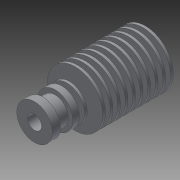
# Autodesk Inventor part: E3D_Chamber
Saved by Autodesk Inventor 2014 (Build 180170000, 170)
## iProperties
Created: 2014-09-30
Part Number: E3D_Chamber
Material: Generic
Document SubType Name: Modeling
Designer: ThatOtherGuy
Density: 1 g/cm^3
Appearance: Default
Author: ThatOtherGuy
Autodesk Inventor part; units mm, degrees
ref_plane "YZ Plane" through (0, 0, 0) normal (1, 0, 0) x (0, 1, 0)
ref_plane "XZ Plane" through (0, 0, 0) normal (0, 1, 0) x (-1, 0, 0)
ref_plane "XY Plane" through (0, 0, 0) normal (0, 0, 1) x (1, 0, 0)
sketch "Sketch1" plane through (0, 0, 0) normal (0, 0, 1) x (1, 0, 0)
  line L0 (0, 0) -> (0, 50.1)
  line L1 (8, 0) -> (8, 3.7)
  line L2 (8, 3.7) -> (6, 3.7)
  line L3 (6, 3.7) -> (6, 9.3)
  line L4 (6, 9.3) -> (8, 9.3)
  line L5 (8, 9.3) -> (8, 12.3)
  line L6 (8, 12.3) -> (4.5, 12.3)
  line L7 (4.5, 12.3) -> (4.5, 14.6)
  line L8 (4.5, 14.6) -> (8, 14.6)
  line L9 (8, 14.6) -> (8, 15.8)
  line L10 (8, 15.8) -> (4.5, 15.8)
  line L11 (4.5, 15.8) -> (4.5, 18.3)
  line L12 (4.5, 18.3) -> (12.5, 18.3)
  line L13 (12.5, 18.3) -> (12.5, 19.5)
  line L14 (12.5, 19.5) -> (4.5, 19.5)
  line L15 (4.5, 19.5) -> (4.5, 21.7)
  line L16 (4.5, 21.7) -> (12.5, 21.7)
  line L17 (12.5, 21.7) -> (12.5, 22.9)
  line L18 (12.5, 22.9) -> (4.5, 22.9)
  line L19 (4.5, 22.9) -> (4.5, 25.1)
  line L20 (4.5, 25.1) -> (12.5, 25.1)
  line L21 (12.5, 25.1) -> (12.5, 26.3)
  line L22 (12.5, 26.3) -> (4.5, 26.3)
  line L23 (4.5, 26.3) -> (4.5, 28.5)
  line L24 (4.5, 28.5) -> (12.5, 28.5)
  line L25 (12.5, 28.5) -> (12.5, 29.7)
  line L26 (12.5, 29.7) -> (6.5, 29.7)
  line L27 (6.5, 29.7) -> (6.5, 31.9)
  line L28 (6.5, 31.9) -> (12.5, 31.9)
  line L29 (12.5, 31.9) -> (12.5, 33.1)
  line L30 (12.5, 33.1) -> (7.5, 33.1)
  line L31 (7.5, 33.1) -> (7.5, 35.3)
  line L32 (7.5, 35.3) -> (12.5, 35.3)
  line L33 (12.5, 35.3) -> (12.5, 36.5)
  line L34 (12.5, 36.5) -> (7.5, 36.5)
  line L35 (7.5, 36.5) -> (7.5, 38.7)
  line L36 (7.5, 38.7) -> (12.5, 38.7)
  line L37 (12.5, 38.7) -> (12.5, 39.9)
  line L38 (12.5, 39.9) -> (7.5, 39.9)
  line L39 (7.5, 39.9) -> (7.5, 42.1)
  line L40 (7.5, 42.1) -> (12.5, 42.1)
  line L41 (12.5, 42.1) -> (12.5, 43.3)
  line L42 (12.5, 43.3) -> (7.5, 43.3)
  line L43 (7.5, 43.3) -> (7.5, 45.5)
  line L44 (7.5, 45.5) -> (12.5, 45.5)
  line L45 (12.5, 45.5) -> (12.5, 46.7)
  line L46 (12.5, 46.7) -> (7.5, 46.7)
  line L47 (7.5, 46.7) -> (7.5, 48.9)
  line L48 (7.5, 48.9) -> (12.5, 48.9)
  line L49 (12.5, 48.9) -> (12.5, 50.1)
  line L50 (12.5, 50.1) -> (3, 50.1)
  line L51 (3, 50.1) -> (3, 32.1)
  line L52 (3, 32.1) -> (1, 31.1)
  line L53 (1, 31.1) -> (1, 19.0785)
  line L54 (1, 19.0785) -> (2, 18.0785)
  line L55 (2, 18.0785) -> (2, 12.0785)
  line L56 (2, 12.0785) -> (3.2, 10)
  line L57 (3.2, 10) -> (3.2, 0)
  line L58 (3.2, 0) -> (8, 0)
  dimension "d2" = 3.7
  dimension "d4" = 16
  dimension "d5" = 12
  dimension "d6" = 9
  dimension "d9" = 3.4
  dimension "d10" = 2.2
  dimension "d11" = 25
  dimension "d12" = 13
  dimension "d13" = 15
  dimension "d16" = 2
  dimension "d17" = 4
  dimension "d18" = 6
  dimension "d21" = 30
  dimension "d22" = 6.4
  dimension "d23" = 10
  dimension "d24" = 6
  dimension "d25" = 18
  dimension "d26" = 1
  dimension "d27" = 50.1
  dimension "d28" = 9.3
  dimension "d29" = 12.3
  dimension "d30" = 14.6
  dimension "d31" = 1
  constraints: 118 end point, 32 parallel, 24 equal length, 19 collinear, 9 perpendicular, 1 coincident, 1 horizontal alignment, 1 vertical
  measures "d2" distance of L1.start L1.end
  measures "d4" diameter of L1 L0
  measures "d5" diameter of L3 L0
  measures "d6" diameter of L7 L0
  measures "d9" distance between parallel lines of L16 L12
  measures "d10" distance between parallel lines of L16 L14
  measures "d11" diameter of L13 L0
  measures "d12" diameter of L27 L0
  measures "d13" diameter of L31 L0
  measures "d16" diameter of L53 L0
  measures "d17" diameter of L55 L0
  measures "d18" diameter of L51 L0
  measures "d21" angle of L57 L56
  measures "d22" diameter of L57 L0
  measures "d23" distance of L57.end L56.end
  measures "d24" distance of L54.end L55.end
  measures "d25" distance of L50.end L51.end
  measures "d26" vertical distance of L51.end L52.end
  measures "d27" distance from line of point (0, 0) L50
  measures "d28" distance between parallel lines of L58 L4
  measures "d29" distance between parallel lines of L58 L6
  measures "d30" distance between parallel lines of L58 L8
  measures "d31" horizontal distance of L53.end L54.end
revolve "Revolution1" add sketch "Sketch1" angle 360 about axis through (0, 0, 0) along (0, 1, 0)
thread "Thread1" size "M6x1" class "6H" standard "ANSI Metric M Profile" length 14 offset 4
body "Solid1"
